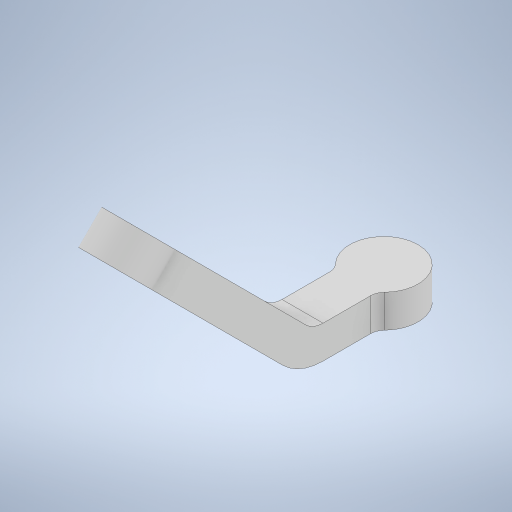
# Autodesk Inventor part: proximal_link_3
Saved by Autodesk Inventor 2024 (Build 280153000, 153)
## iProperties
Created: 2023-10-30
Part Number: proximal_link_3
Material: Generic
Document SubType Name: Modeling
Designer: MATEO
Density: 1 g/cm^3
Appearance: Default
Author: MATEO
Autodesk Inventor part; units mm, degrees
ref_plane "YZ Plane" through (0, 0, 0) normal (1, 0, 0) x (0, 1, 0)
ref_plane "XZ Plane" through (0, 0, 0) normal (0, 1, 0) x (-1, 0, 0)
sketch "Sketch1" plane through (0, 0, 0) normal (0, 1, 0) x (-1, 0, 0)
  arc A0 (-8.928571, 8.748178) -> (8.928571, 8.748178) centre (0, 0) ccw
  line L0 (-7.5, 12.247449) -> (-7.5, 20)
  line L1 (7.5, 20) -> (7.5, 12.247449)
  line L2 (7.5, 20) -> (-7.5, 20)
  arc A1 (7.5, 12.247449) -> (8.928571, 8.748178) centre (12.5, 12.247449) ccw
  arc A2 (-8.928571, 8.748178) -> (-7.5, 12.247449) centre (-12.5, 12.247449) ccw
  point P0 (7.5, 10)
  point P1 (-7.5, 10)
  point P2 (0, 10)
  point P3 (0, 20)
  dimension "d0" = 25
  dimension "d106" = 15
  dimension "d107" = 10
  dimension "d108" = 10
  dimension "d109" = 5
  constraints: 8 point on circle, 6 end point, 4 tangent, 3 centre point, 2 horizontal alignment, 2 point on line, 2 vertical alignment, 1 coincident, 1 equal radius, 1 midpoint, 1 parallel
  measures "d0" diameter of A0
  measures "d106" distance of L0.end L1.start
  measures "d107" distance of point (-7.5, 10) L0.end
  measures "d108" distance of point (0, 10) point (0, 0)
  measures "d109" radius of A1
extrude "Extrusion1" add sketch "Sketch1" against normal blind 12
sketch "Sketch22" plane through (-7.5, 0, 20) normal (0, 0, 1) x (1, 0, 0)
  line L0 (0, 0) -> (0, -12) projected
  line L1 (15, -12) -> (0, -12) projected
  line L2 (0, 0) -> (15, 0)
  line L3 (15, 0) -> (15, -12)
  line L4 (15, -12) -> (0, -12)
  line L5 (0, -12) -> (0, 0)
  point P0 (7.5, 0)
  constraints: 8 end point, 2 parallel, 1 horizontal, 1 perpendicular
sketch "Sketch23" plane through (0, 0, 0) normal (1, 0, 0) x (0, 1, 0)
  line L0 (0, 20) -> (-12, 20)
  line L1 (-6, 20) -> (-6, 29.70611)
  line L2 (-1.606602, 40.312712) -> (43.497475, 85.416788)
  arc A0 (-1.606602, 40.312712) -> (-6, 29.70611) centre (9, 29.70611) ccw
  point P0 (0, 0)
  point P1 (-6, 35.919313)
  dimension "d110" = 15.91931
  dimension "d111" = 70
  dimension "d112" = 135
  dimension "d113" = 15
  constraints: 4 end point, 2 point on circle, 2 point on line, 2 tangent, 1 centre point, 1 midpoint, 1 vertical
  measures "d110" distance of L1.start point (-6, 35.919)
  measures "d111" distance of point (-6, 35.919) L2.end
  measures "d112" angle of L1 L2
  measures "d113" radius of A0
sweep "Sweep2" add profiles "Sketch22" path "Sketch23" path curves L1 A0 L2
ref_plane "Work Plane11" through (7.5, -1.606602, 40.312712) normal (0, 0.7071068, -0.7071068) x (-1, 0, 0)
sketch "Sketch24" plane through (7.5, -1.606602, 40.312712) normal (0, 0.7071068, -0.7071068) x (-1, 0, 0)
  line L0 (0, 63.786797) -> (15, 63.786797)
  line L1 (0, 63.786797) -> (15, 63.786797)
  line L2 (0, 63.786797) -> (0, 67.740058)
  line L3 (15, 63.786797) -> (15, 67.740058)
  arc A0 (15, 67.740058) -> (0, 67.740058) centre (7.5, 75.786797) ccw
  line L4 (0, 63.786797) -> (15, 63.786797)
  point P0 (7.5, -27.369353)
  point P1 (7.5, 63.786797)
  point P2 (7.5, 63.786797)
  dimension "d129" = 22
  dimension "d130" = 12
  constraints: 8 end point, 2 horizontal alignment, 2 midpoint, 2 point on circle, 2 vertical, 1 centre point, 1 collinear, 1 vertical alignment
  measures "d129" diameter of A0
  measures "d130" distance from line of L0 A0.centre
extrude "Extrusion17" add sketch "Sketch24" along normal mid plane 12
sketch "Sketch25" plane through (-7.5, -5.849242, 44.555352) normal (0, -0.7071068, 0.7071068) x (1, 0, 0)
  circle A0 centre (7.5, 75.786797) radius 2.5
  arc A1 (15, 67.740058) -> (0, 67.740058) centre (7.5, 75.786797) ccw
  point P0 (7.5, -27.369353)
  dimension "d123" = 5
  constraints: 2 coincident, 1 centre point
  measures "d123" diameter of A0
extrude "Extrusion18" cut sketch "Sketch25" against normal through all
sketch "Sketch26" plane through (0, -12, 0) normal (0, -1, 0) x (1, 0, 0)
  circle A0 centre (0, 0) radius 7.6
  dimension "d126" = 15.2
  constraints: 1 centre point, 1 coincident
  measures "d126" diameter of A0
extrude "Extrusion19" cut sketch "Sketch26" against normal blind 5
sketch "Sketch27" plane through (7.5, 2.636039, 36.070071) normal (0, 0.7071068, -0.7071068) x (-1, 0, 0)
  circle A0 centre (7.5, 75.786797) radius 2.5
  circle A1 centre (7.5, 75.786797) radius 8.1
  point P0 (7.5, -27.369353)
  dimension "d131" = 16.2
  constraints: 1 centre point, 1 coincident
  measures "d131" diameter of A1
extrude "Extrusion20" cut sketch "Sketch27" against normal blind 5
mirror "Mirror2" about plane through (7.5, -1.606602, 40.312712) normal (0, 0.7071068, -0.7071068) of "Extrusion20"
body "Solid1"
